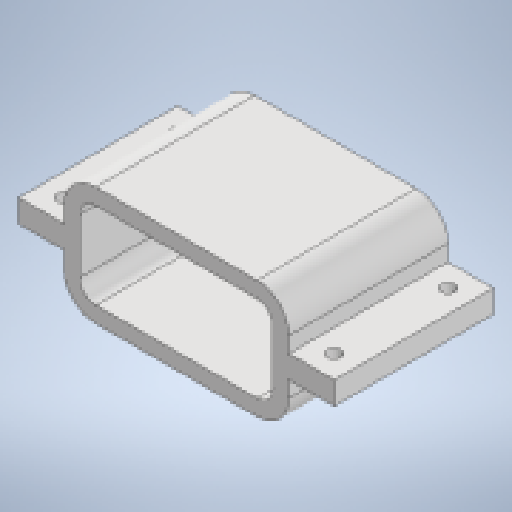
# Autodesk Inventor part: camHolder
Saved by Autodesk Inventor 2025.1 (Build 291241000, 241)
## iProperties
Created: 2025-06-16
Part Number: camHolder
Material: Generic
Document SubType Name: Modeling
Designer: User
Density: 1 g/cm^3
Appearance: Default
Author: User
Autodesk Inventor part; units mm, degrees
ref_plane "YZ Plane" through (0, 0, 0) normal (1, 0, 0) x (0, 1, 0)
ref_plane "XZ Plane" through (0, 0, 0) normal (0, 1, 0) x (-1, 0, 0)
ref_plane "XY Plane" through (0, 0, 0) normal (0, 0, 1) x (1, 0, 0)
sketch "Sketch1" plane through (0, 0, 0) normal (0, 0, 1) x (1, 0, 0)
  arc A0 (0, -3) -> (3, 0) centre (0, 0) ccw projected
  line L0 (3, 12) -> (3, 0) projected
  arc A1 (3, 12) -> (0, 15) centre (0, 12) ccw projected
  line L1 (-34, 15) -> (0, 15) projected
  arc A2 (-34, 15) -> (-37, 12) centre (-34, 12) ccw projected
  line L2 (-37, 0) -> (-37, 12) projected
  arc A3 (-37, 0) -> (-34, -3) centre (-34, 0) ccw projected
  line L3 (0, -3) -> (-34, -3) projected
  arc A4 (-32.9749, 5.5) -> (-28, 1) centre (-28, 6) ccw projected
  arc A5 (-28, 10) -> (-32.9749, 5.5) centre (-28, 5) ccw projected
  line L4 (-6, 10) -> (-28, 10) projected
  arc A6 (-1.0251, 5.5) -> (-6, 10) centre (-6, 5) ccw projected
  arc A7 (-6, 1) -> (-1.0251, 5.5) centre (-6, 6) ccw projected
  line L5 (-28, 1) -> (-6, 1) projected
  line L6 (-37.75, 0) -> (-37.75, 12)
  line L7 (3.75, 12) -> (3.75, 0)
  line L8 (0, 0) -> (0.75, 0)
  line L9 (0, 12) -> (0.75, 12)
  line L10 (-34, 12) -> (-34.75, 12)
  line L11 (-34, 0) -> (-34.75, 0)
  arc A8 (-37.75, 0) -> (-34.75, -3) centre (-34.75, 0) ccw
  line L12 (-34.75, 0) -> (-34.75, -3) construction
  line L13 (-34.75, 0) -> (-31.75, 0) construction
  arc A9 (0.75, -3) -> (3.75, 0) centre (0.75, 0) ccw
  arc A10 (3.75, 12) -> (0.75, 15) centre (0.75, 12) ccw
  arc A11 (-34.75, 15) -> (-37.75, 12) centre (-34.75, 12) ccw
  line L14 (-34.75, 12) -> (-34.75, 15) construction
  line L15 (-34.75, 12) -> (-37.75, 12) construction
  line L16 (-34, -3) -> (-34.75, -3)
  line L17 (-34, 15) -> (-34.75, 15)
  line L18 (0, 15) -> (0.75, 15)
  line L19 (0, -3) -> (0.75, -3)
  line L20 (-34, 15) -> (0, 15)
  line L21 (-34, -3) -> (0, -3)
  line L22 (-38.25, 12) -> (-38.25, 0)
  arc A12 (-38.25, 0) -> (-34.75, -3.5) centre (-34.75, 0) ccw
  line L23 (-34.75, -3.5) -> (-34, -3.5)
  line L24 (-34, -3.5) -> (0, -3.5)
  line L25 (0, -3.5) -> (0.75, -3.5)
  arc A13 (0.75, -3.5) -> (4.25, 0) centre (0.75, 0) ccw
  line L26 (4.25, 0) -> (4.25, 12)
  arc A14 (4.25, 12) -> (0.75, 15.5) centre (0.75, 12) ccw
  line L27 (0.75, 15.5) -> (0, 15.5)
  line L28 (0, 15.5) -> (-34, 15.5)
  line L29 (-34, 15.5) -> (-34.75, 15.5)
  arc A15 (-34.75, 15.5) -> (-38.25, 12) centre (-34.75, 12) ccw
  line L30 (-41.75, 12) -> (-41.75, 0)
  arc A16 (-41.75, 0) -> (-34.75, -7) centre (-34.75, 0) ccw
  line L31 (-34.75, -7) -> (-34, -7)
  line L32 (-34, -7) -> (0, -7)
  line L33 (0, -7) -> (0.75, -7)
  arc A17 (0.75, -7) -> (7.75, 0) centre (0.75, 0) ccw
  line L34 (7.75, 0) -> (7.75, 12)
  arc A18 (7.75, 12) -> (0.75, 19) centre (0.75, 12) ccw
  line L35 (0.75, 19) -> (0, 19)
  line L36 (0, 19) -> (-34, 19)
  line L37 (-34, 19) -> (-34.75, 19)
  arc A19 (-34.75, 19) -> (-41.75, 12) centre (-34.75, 12) ccw
  point P0 (0, 0)
  dimension "d1" = 40
  dimension "d4" = 0.75
  dimension "d5" = 0.75
  dimension "d6" = 0.75
  dimension "d7" = 0.75
  dimension "d8" = 0.75
  dimension "d9" = 90
  dimension "d10" = 90
  dimension "d11" = 0.5
  dimension "d12" = 3.5
  constraints: 65 end point, 24 point on circle, 12 centre point, 6 horizontal, 4 coincident, 3 parallel, 3 tangent, 1 perpendicular, 22 other
  measures "d1" distance between parallel lines of L0 L2
  measures "d4" distance of L7.end L0.end
  measures "d5" distance of L8.start L8.end
  measures "d6" distance of L9.start L9.end
  measures "d7" distance of L10.start L10.end
  measures "d8" distance of L11.start L11.end
  measures "d9" angle of L12 L13
  measures "d10" angle of L14 L15
  measures "d11" radial gap between concentric circles of A11 A15
  measures "d12" radial gap between concentric circles of A15 A19
extrude "Extrusion1" add sketch "Sketch1" against normal blind 35 contours A19 L37 L36 L35 A18 L34 A17 L33 L32 L31 A16 L30
sketch "Sketch2" plane through (0, 0, 0) normal (0, 0, 1) x (1, 0, 0)
  line L0 (-41.75, 12) -> (-41.75, 0) projected
  line L1 (7.75, 0) -> (7.75, 12) projected
  line L2 (7.75, 6) -> (17.75, 6)
  line L3 (-41.75, 6) -> (-51.75, 6)
  line L4 (-41.75, 8.5) -> (-51.75, 8.5)
  line L5 (-41.75, 3.5) -> (-51.75, 3.5)
  line L6 (7.75, 8.5) -> (17.75, 8.5)
  line L7 (7.75, 3.5) -> (17.75, 3.5)
  line L8 (17.75, 8.5) -> (7.75, 8.5)
  line L9 (7.75, 8.5) -> (7.75, 3.5)
  line L10 (7.75, 3.5) -> (17.75, 3.5)
  line L11 (17.75, 3.5) -> (17.75, 8.5)
  line L12 (-51.75, 8.5) -> (-41.75, 8.5)
  line L13 (-41.75, 8.5) -> (-41.75, 3.5)
  line L14 (-41.75, 3.5) -> (-51.75, 3.5)
  line L15 (-51.75, 3.5) -> (-51.75, 8.5)
  point P0 (0, 0)
  dimension "d15" = 10
  dimension "d16" = 10
  dimension "d17" = 2.5
  dimension "d18" = 2.5
  dimension "d19" = 2.5
  dimension "d20" = 2.5
  constraints: 28 end point, 8 parallel, 4 horizontal, 2 midpoint, 2 perpendicular
  measures "d15" distance of L2.start L2.end
  measures "d16" distance of L3.start L3.end
  measures "d17" distance between parallel lines of L3 L4
  measures "d18" distance between parallel lines of L3 L5
  measures "d19" distance between parallel lines of L2 L6
  measures "d20" distance between parallel lines of L2 L7
extrude "Extrusion2" add sketch "Sketch2" against normal up to surface (35 mm away)
sketch "Sketch3" plane through (7.75, 3.5, 0) normal (0, -1, 0) x (1, 0, 0)
  line L0 (10, -35) -> (0, -35) projected
  line L1 (10, 0) -> (10, -35) projected
  line L2 (0, 0) -> (10, 0) projected
  line L3 (0, -35) -> (0, 0) projected
  line L4 (-49.5, -35) -> (-59.5, -35) projected
  line L5 (-49.5, 0) -> (-49.5, -35) projected
  line L6 (-59.5, 0) -> (-49.5, 0) projected
  line L7 (-59.5, 0) -> (-59.5, -35) projected
  circle A0 centre (5, -5) radius 5
  circle A1 centre (5, -30) radius 5
  circle A2 centre (-54.5, -5) radius 5
  circle A3 centre (-54.5, -30) radius 5
  circle A4 centre (-54.5, -5) radius 1.5
  circle A5 centre (-54.5, -30) radius 1.5
  circle A6 centre (5, -5) radius 1.5
  circle A7 centre (5, -30) radius 1.5
  point P0 (-7.75, 0)
  dimension "d23" = 3
  dimension "d24" = 3
  dimension "d25" = 3
  dimension "d26" = 3
  constraints: 12 tangent, 8 centre point, 4 coincident
  measures "d23" diameter of A4
  measures "d24" diameter of A5
  measures "d25" diameter of A6
  measures "d26" diameter of A7
extrude "Extrusion3" cut sketch "Sketch3" against normal blind 10 contours A4 | A5 | A6 | A7
sketch "Sketch4" plane through (-34.75, -7, 0) normal (0, -1, 0) x (1, 0, 0)
  line L0 (0, 0) -> (35.5, 0) projected
  line L1 (17.75, 0) -> (17.75, -26)
  line L2 (17.75, -26) -> (17.75, -31)
  circle A0 centre (17.75, -28.5) radius 2.5
  circle A1 centre (17.75, -28.5) radius 1.4
  point P0 (34.75, 0)
  dimension "d29" = 26
  dimension "d30" = 5
  dimension "d31" = 2.8
  constraints: 4 end point, 2 midpoint, 2 vertical, 1 centre point, 1 coincident, 1 vertical alignment, 2 other
  measures "d29" distance of L1.start L1.end
  measures "d30" distance of L1.end L2.end
  measures "d31" diameter of A1
extrude "Extrusion4" cut sketch "Sketch4" against normal blind 10 contours A1 L2 | L2 A1
equation "\"d21\" = d18"
body "Solid1"
